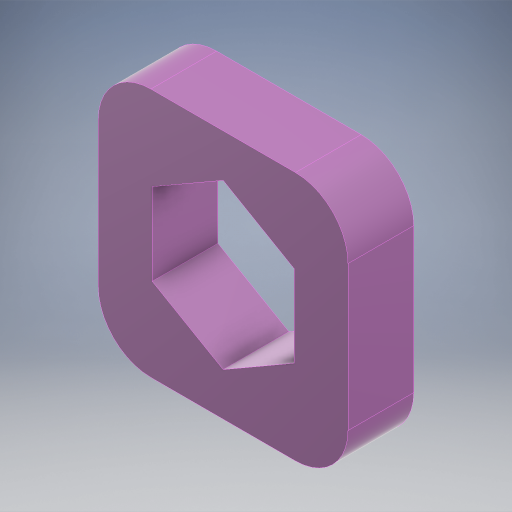
# Autodesk Inventor part: М3 вставка
Saved by Autodesk Inventor 2023 (Build 270158000, 158)
## iProperties
Created: 2023-03-26
Part Number: М3 вставка
Material: Типовые
Document SubType Name: Modeling
Designer: Admin
Density: 1 g/cm^3
Appearance: По умолчанию
Author: Admin
Autodesk Inventor part; units mm, degrees
ref_plane "YZ Plane" through (0, 0, 0) normal (1, 0, 0) x (0, 1, 0)
ref_plane "XZ Plane" through (0, 0, 0) normal (0, 1, 0) x (-1, 0, 0)
ref_plane "XY Plane" through (0, 0, 0) normal (0, 0, 1) x (1, 0, 0)
sketch "Эскиз1" plane through (0, 0, 0) normal (0, 0, 1) x (1, 0, 0)
  arc A0 (-2.75, 4.75) -> (-4.75, 2.75) centre (-2.75, 2.75) ccw
  line L0 (-2.7, 1.5588) -> (0, 3.1177)
  line L1 (-2.7, -1.5588) -> (-2.7, 1.5588)
  line L2 (-4.75, 2.75) -> (-4.75, -2.75)
  line L3 (2.75, 4.75) -> (-2.75, 4.75)
  line L4 (0, 3.1177) -> (2.7, 1.5588)
  line L5 (0, -3.1177) -> (-2.7, -1.5588)
  arc A1 (4.75, 2.75) -> (2.75, 4.75) centre (2.75, 2.75) ccw
  line L6 (2.7, 1.5588) -> (2.7, -1.5588)
  line L7 (-4.75, -4.75) -> (4.75, 4.75) construction
  line L8 (4.75, -4.75) -> (-4.75, 4.75) construction
  line L9 (4.75, -2.75) -> (4.75, 2.75)
  line L10 (-2.75, -4.75) -> (2.75, -4.75)
  line L11 (2.7, -1.5588) -> (0, -3.1177)
  arc A2 (2.75, -4.75) -> (4.75, -2.75) centre (2.75, -2.75) ccw
  arc A3 (-4.75, -2.75) -> (-2.75, -4.75) centre (-2.75, -2.75) ccw
  point P0 (0, 0)
  point P1 (0, 0)
  dimension "d1" = 2
  dimension "d2" = 2
  constraints: 24 end point, 8 point on circle, 8 point on line, 8 tangent, 4 centre point, 4 parallel, 2 equal radius, 2 midpoint, 2 perpendicular, 1 coincident, 1 horizontal, 1 vertical, 13 other
  measures "d1" radius of A0
  measures "d2" radius of A2
extrude "Выдавливание1" add sketch "Эскиз1" along normal blind 2.5
